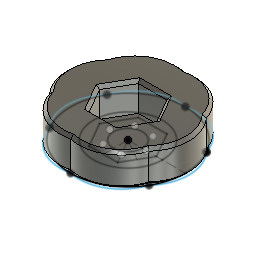
Bolt Thumbscrew Wide-Flat (Autodesk Fusion 360 design; units mm, degrees)
Autodesk Fusion 360 part; units mm, degrees
sketch "Sketch1" plane through (0, 0, 0) normal (0, 0, 1) x (1, 0, 0)
  circle A0 centre (0, 0) radius 3.175
  line L0 (3.1529, 5.461) -> (-3.1529, 5.461)
  line L1 (-3.1529, 5.461) -> (-6.3058, 0)
  line L2 (-6.3058, 0) -> (-3.1529, -5.461)
  line L3 (-3.1529, -5.461) -> (3.1529, -5.461)
  line L4 (3.1529, -5.461) -> (6.3058, 0)
  line L5 (6.3058, 0) -> (3.1529, 5.461)
  circle A1 centre (0, 0) radius 12.7
  line L6 (0, 0) -> (12.7, 0) construction
  line L7 (0, 0) -> (3.1529, -5.461) construction
  line L8 (0, 0) -> (4.7294, -2.7305) construction
  line L9 (0, 0) -> (0, -5.461) construction
  arc A2 (0, -12.7) -> (10.9985, -6.35) centre (2.0207, -3.5) ccw
  arc A3 (10.9985, -6.35) -> (10.9985, 6.35) centre (4.0415, 0) ccw
  arc A4 (10.9985, 6.35) -> (0, 12.7) centre (2.0207, 3.5) ccw
  arc A5 (0, 12.7) -> (-10.9985, 6.35) centre (-2.0207, 3.5) ccw
  arc A6 (-10.9985, 6.35) -> (-10.9985, -6.35) centre (-4.0415, 0) ccw
  arc A7 (-10.9985, -6.35) -> (0, -12.7) centre (-2.0207, -3.5) ccw
  circle A8 centre (0, 0) radius 7.62
  dimension "d1" = 6.35
  dimension "d2" = 5.461
  dimension "d13" = 360
  dimension "d16" = 25.4
  dimension "d17" = 15.24
  constraint coincident A0.centre A1.centre
  constraint horizontal L0
  constraint coincident A1 L6.end
  constraint horizontal L6
  constraint midpoint L4 L8.end
  constraint midpoint L3 L9.end
  constraint coincident A1 A2.end
  constraint coincident A1 A2.start
  constraint coincident L9 A2.start
  constraint coincident L8 A2.end
  measures "d1" diameter of A0
  measures "d2" distance of A0.centre L5
  measures "d16" diameter of A1
  measures "d17" diameter of A8
extrude "Extrude1" add sketch "Sketch1" along normal blind 0.8 contours L0 L1 L2 L3 L4 L5 | A1 | A1 A3 | A1 A4 | A1 A2 | A1 A5 | A1 A7 | A1 A6 | A8
extrude "Extrude2" add sketch "Sketch1" along normal blind 6.35 from surface at 0.8 contours A1 | A1 A3 | A1 A4 | A1 A2 | A1 A5 | A1 A7 | A1 A6 | A8
extrude "Extrude3" add sketch "Sketch1" against normal blind 2.54 contours L0 L1 L2 L3 L4 L5 | A8
extrude "Extrude4" add sketch "Sketch1" against normal blind 0.3 from surface at 0.8 contours A0
chamfer "Chamfer1" distance 0.635 angle 45 3 faces at (-6.8191, 3.937, 7.15) (-5.3389, 10.173, 0) (6.0981, -0.5363, -2.54)
equation "d2 = ( 0.43 / 2 ) * 1 in"
